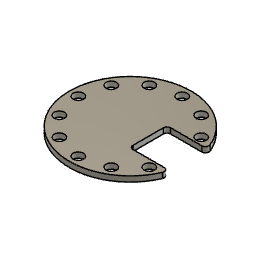
cryo head clamp v8 (Autodesk Fusion 360 design; units mm, degrees)
Autodesk Fusion 360 part; units mm, degrees
note: some values were not read from the file. Set by a fixed rule: the direction of a hole.
sketch "Sketch1" plane through (0, 0, 0) normal (0, 1, 0) x (1, 0, 0)
  circle A0 centre (0, 0) radius 29 construction
  circle A1 centre (0, 0) radius 34
  line L0 (32.3381, 10.5) -> (10, 10.5)
  line L1 (10, 10.5) -> (10, -10.5)
  line L2 (10, -10.5) -> (32.3381, -10.5)
  point P0 (0, 29)
  dimension "d1" = 58
  dimension "d2" = 68
  dimension "d3" = 21
  dimension "d4" = 10
  constraint coincident A0.centre A1.centre
  constraint concentric A0 A1
  constraint coincident A1 L0.start
  constraint horizontal L0
  constraint perpendicular L0 L1
  constraint coincident A1 L2.end
  constraint perpendicular L1 L2
  constraint vertical L0.start L2.end
  constraint coincident A0 P0
  constraint vertical A0.centre P0
  measures "d1" diameter of A0
  measures "d2" diameter of A1
  measures "d3" distance of L0 L2
  measures "d4" distance of A0.centre L1
extrude "Extrude1" add sketch "Sketch1" along normal blind 3 contours A1 L0 L1 L2 picked at (-4.6667, 0)
hole "Hole1" at (0, 0, -29) direction (0, 1, 0) diameter 5.8 depth 3 tip angle 118
pattern_circular "C-Pattern1" count 12 over 360 about axis through (0, 1.75, 0) along (0, 1, 0) of "Hole1"
fillet "Fillet1" radius 2 4 edges at (10, 1.5, -10.5) (10, 1.5, 10.5) (32.3381, 1.5, -10.5) (32.3381, 1.5, 10.5)
sketch "Sketch2" plane through (0, 3, 0) normal (0, 1, 0) x (-1, 0, 0)
  circle A0 centre (-14.5, -25.1147) radius 2.9
  circle A1 centre (-14.5, 25.1147) radius 2.9
  circle A2 centre (0, 29) radius 2.9
  circle A3 centre (14.5, 25.1147) radius 2.9
  circle A4 centre (25.1147, 14.5) radius 2.9
  circle A5 centre (29, 0) radius 2.9
  circle A6 centre (25.1147, -14.5) radius 2.9
  circle A7 centre (14.5, -25.1147) radius 2.9
  circle A8 centre (0, -29) radius 2.9
  arc A9 (-31.2987, 13.2812) -> (-29.4576, 10.5) centre (-29.4576, 12.5) ccw
  line L0 (-29.4576, 10.5) -> (-12, 10.5)
  arc A10 (-10, 8.5) -> (-12, 10.5) centre (-12, 8.5) ccw
  line L1 (-10, 8.5) -> (-10, -8.5)
  arc A11 (-12, -10.5) -> (-10, -8.5) centre (-12, -8.5) ccw
  line L2 (-12, -10.5) -> (-29.4576, -10.5)
  arc A12 (-29.4576, -10.5) -> (-31.2987, -13.2813) centre (-29.4576, -12.5) ccw
  arc A13 (-31.2987, -13.2813) -> (-31.2987, 13.2813) centre (0, 0) ccw
  circle A14 centre (-25.1147, -14.5) radius 2.9
  circle A15 centre (-25.1147, 14.5) radius 2.9
